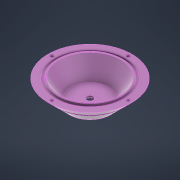
# Autodesk Inventor part: 001
Saved by Autodesk Inventor 2022 (Build 260153000, 153)
## iProperties
Created: 2021-10-30
Part Number: 001
Material: Iron, Cast
Document SubType Name: Modeling
Designer: vinicius.miguel
Density: 7.15 g/cm^3
Appearance: Smooth - Purple
Mass: 117.151 g
Surface Area: 93.5686 cm^2
Volume: 14.9237 cm^3
Author: vinicius.miguel
Autodesk Inventor part; units mm, degrees
ref_plane "YZ Plane" through (0, 0, 0) normal (1, 0, 0) x (0, 1, 0)
ref_plane "XZ Plane" through (0, 0, 0) normal (0, 1, 0) x (-1, 0, 0)
ref_plane "XY Plane" through (0, 0, 0) normal (0, 0, 1) x (1, 0, 0)
sketch "Sketch1" plane through (0, 0, 0) normal (0, 0, 1) x (1, 0, 0)
  line L0 (4.5, 0) -> (16.2, 0)
  line L1 (32.5, 16.3) -> (27, 16.3)
  line L2 (27, 16.3) -> (27, 15.07)
  line L3 (27, 15.07) -> (25, 15.07)
  line L4 (15, 3) -> (2.5, 3)
  line L5 (2.5, 3) -> (2.5, 2)
  line L6 (0, 0) -> (0, 9.8768)
  line L7 (2.5, 2) -> (4.5, 0)
  line L8 (15, 3) -> (23.7482, 17)
  line L9 (23.7482, 17) -> (25, 17)
  line L10 (25, 17) -> (25, 15.07)
  line L11 (16.2, 0) -> (25, 8.8)
  line L12 (25, 8.8) -> (25, 10.8)
  line L13 (25, 10.8) -> (27, 10.8)
  line L14 (27, 10.8) -> (32.5, 16.3)
  point P0 (2.5, 0)
  dimension "d0" = 5
  dimension "d1" = 3
  dimension "d11" = 2
  dimension "d12" = 2
  dimension "d20" = 17
  dimension "d22" = 16.3
  dimension "d23" = 50
  dimension "d24" = 1.23
  dimension "d25" = 2
  dimension "d26" = 30
  dimension "d28" = 65
  dimension "d29" = 5.5
  dimension "d30" = 50
  dimension "d42" = 135
  dimension "d43" = 32
  constraints: 30 end point, 4 perpendicular, 2 horizontal, 2 parallel, 2 point on line, 2 vertical, 1 collinear, 1 horizontal alignment
  measures "d0" diameter of L5 L6
  measures "d1" distance of L4.end point (2.5, 0)
  measures "d11" distance of L5.end point (2.5, 0)
  measures "d12" distance of L0.start point (2.5, 0)
  measures "d20" distance from line of L9 L6.start
  measures "d22" distance from line of L1 L6.start
  measures "d23" diameter of L10 L6
  measures "d24" distance of L1.end L2.end
  measures "d25" distance of L2.end L3.end
  measures "d26" diameter of L4.start L6
  measures "d28" diameter of L1.start L6
  measures "d29" distance between parallel lines of L13 L1
  measures "d30" diameter of L12 L6
  measures "d42" angle of L0 L11
  measures "d43" angle of L8 L6
revolve "Revolution1" add sketch "Sketch1" angle 360 about axis through (0, 0, 0) along (0, 1, 0)
sketch "Sketch2" plane through (0, 10.8, 0) normal (0, -1, 0) x (1, 0, 0)
  point P0 (0, 0)
  point P1 (29.5, 0)
  dimension "d38" = 29.5
  measures "d38" distance of point (29.5, 0) point (0, 0)
hole "Hole1" at (29.5, 10.8, 0) direction (0, 1, 0) diameter 2.4 end through all counterbore diameter 4.4 counterbore depth 4.5 clearance for "Socket Head Cap Screw ISO 4762" size "M2" standard "ISO"
pattern_circular "Circular Pattern1" count 4 over 360 about axis through (0, -10, 0) along (0, 1, 0) of "Hole1"
equation "\"d12\" = d11"
body "Solid1"
